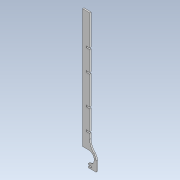
# Autodesk Inventor part: chassis_1_5
Saved by Autodesk Inventor 2022 (Build 260153000, 153)
## iProperties
Created: 2023-04-28
Part Number: chassis_1_5
Material: 一般
Document SubType Name: Modeling
Designer: Johnny Jou
Density: 1 g/cm^3
Appearance: 預設
Author: Johnny Jou
Autodesk Inventor part; units mm, degrees
ref_plane "YZ Plane" through (0, 0, 0) normal (1, 0, 0) x (0, 1, 0)
ref_plane "XZ Plane" through (0, 0, 0) normal (0, 1, 0) x (-1, 0, 0)
ref_plane "XY Plane" through (0, 0, 0) normal (0, 0, 1) x (1, 0, 0)
sketch "草圖1" plane through (0, 0, 0) normal (0, 0, 1) x (1, 0, 0)
  arc A0 (-7.5, 147.4544) -> (-7.5, 136.5456) centre (-10, 142) ccw construction
  arc A1 (-10, 4.5) -> (1.3043, 31.8231) centre (-10, 20.5) ccw
  line L0 (-10, 20.5) -> (-10, 4.5) construction
  line L1 (-10, 20.5) -> (-10, 48.1702) construction
  line L2 (-10, 8.3) -> (-10, 4.5)
  line L3 (-7.5, 284) -> (-22.5, 284)
  line L4 (-22.5, 284) -> (-22.5, 48.1702)
  line L5 (-22.5, 48.1702) -> (-10, 48.1702) construction
  line L6 (-7.5, 36.5) -> (-7.5, 53.0538) construction
  line L7 (-7.5, 36.5) -> (-7.5, 36.3035) construction
  line L8 (-10, 48.1702) -> (-10, 32.7) construction
  line L9 (-10, 32.7) -> (-22.5, 32.7)
  line L10 (-22.5, 32.7) -> (-22.5, 48.1702)
  arc A2 (-7.5, 53.0538) -> (1.3043, 31.8231) centre (22.5, 53.0538) ccw
  arc A3 (1.3043, 31.8231) -> (-7.5, 36.3035) centre (-10, 20.5) ccw construction
  line L11 (-7.5, 53.0538) -> (-7.5, 64.05)
  line L12 (-7.5, 219.95) -> (-15, 219.95)
  line L13 (-15, 219.95) -> (-15, 217)
  line L14 (-15, 217) -> (-7.5, 217)
  line L15 (-7.5, 217) -> (-7.5, 219.95) construction
  line L16 (-7.5, 174.95) -> (-15, 174.95)
  line L17 (-15, 174.95) -> (-15, 172)
  line L18 (-15, 172) -> (-7.5, 172)
  line L19 (-7.5, 172) -> (-7.5, 174.95) construction
  line L20 (-7.5, 112) -> (-15, 112)
  line L21 (-15, 112) -> (-15, 109.05)
  line L22 (-15, 109.05) -> (-7.5, 109.05)
  line L23 (-7.5, 109.05) -> (-7.5, 112) construction
  line L24 (-7.5, 67) -> (-15, 67)
  line L25 (-15, 67) -> (-15, 64.05)
  line L26 (-15, 64.05) -> (-7.5, 64.05)
  line L27 (-7.5, 64.05) -> (-7.5, 67) construction
  line L28 (-7.5, 217) -> (-7.5, 219.95) construction
  line L29 (-7.5, 174.95) -> (-7.5, 217)
  line L30 (-7.5, 172) -> (-7.5, 174.95) construction
  line L31 (-7.5, 112) -> (-7.5, 172)
  line L32 (-7.5, 109.05) -> (-7.5, 112) construction
  line L33 (-7.5, 67) -> (-7.5, 109.05)
  line L34 (-7.5, 64.05) -> (-7.5, 67) construction
  line L35 (-7.5, 219.95) -> (-7.5, 284)
  arc A4 (-10, 8.3) -> (-10, 32.7) centre (-10, 20.5) ccw
  arc A5 (-12.7221, 32.7) -> (-10, 8) centre (-10, 20.5) ccw construction
  line L36 (-10, 4.5) -> (6, 4.5)
  line L37 (6, 4.5) -> (6, 0)
  line L38 (6, 0) -> (-10, 0)
  line L39 (-10, 0) -> (-10, 4.5)
  line L40 (6, 4.5) -> (6, 20.5)
  point P0 (0, 0)
  dimension "d12" = 16
  dimension "d13" = 180
  dimension "d14" = 15
  dimension "d16" = 60
  dimension "d17" = 30
  dimension "d18" = 75
  dimension "d19" = 30
  dimension "d20" = 75
  dimension "d21" = 2.95
  dimension "d22" = 2.95
  dimension "d23" = 2.95
  dimension "d24" = 2.95
  dimension "d25" = 7.5
  dimension "d30" = 24.4
  dimension "d31" = 25
  dimension "d32" = 4.5
  dimension "d38" = 284
  constraints: 82 end point, 20 parallel, 13 point on circle, 13 tangent, 11 point on line, 8 perpendicular, 7 horizontal, 6 centre point, 2 coincident, 2 collinear, 2 vertical, 3 other
  measures "d12" radius of A1
  measures "d13" angle of L0 L1
  measures "d14" distance between parallel lines of L4 L6
  measures "d16" diameter of A2
  measures "d17" distance from line of L20 A0.centre
  measures "d18" distance from line of L24 A0.centre
  measures "d19" distance from line of L18 A0.centre
  measures "d20" distance from line of L14 A0.centre
  measures "d21" distance of L16.end L17.end
  measures "d22" distance of L12.end L13.end
  measures "d23" distance of L20.end L21.end
  measures "d24" distance of L24.end L25.end
  measures "d25" distance between parallel lines of L11 L25
  measures "d30" diameter of A4
  measures "d31" diameter of A5
  measures "d32" distance of L36.end L37.end
  measures "d38" distance between parallel lines of L3 L38
extrude "擠出1" add sketch "草圖1" along normal blind 3
sketch "草圖3" plane through (0, 0, 3) normal (0, 0, 1) x (1, 0, 0)
  line L0 (-10, 8.3) -> (-10, 0) projected
  line L1 (-10, 5.9) -> (-4, 5.9)
  line L2 (-4, 5.9) -> (-4, 3)
  line L3 (-4, 3) -> (-10, 3)
  line L4 (-10, 3) -> (-10, 5.9)
  line L5 (-10, 0) -> (6, 0) projected
  point P0 (0, 0)
  dimension "d33" = 2.9
  dimension "d34" = 3
  dimension "d35" = 6
  constraints: 8 end point, 2 parallel, 1 horizontal, 1 perpendicular, 1 point on line
  measures "d33" distance between parallel lines of L3 L1
  measures "d34" distance between parallel lines of L5 L3
  measures "d35" distance between parallel lines of L0 L2
extrude "擠出2" cut sketch "草圖3" against normal up to surface (3 mm away)
equation "\"d25\" = 0.5 * d14"
